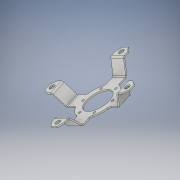
# Autodesk Inventor part: Actividad 4.1_Emily_Rojas
Saved by Autodesk Inventor 2019 (Build 230136000, 136)
## iProperties
Created: 2019-05-23
Part Number: Actividad 4.1_Emily_Rojas
Material: Generic
Document SubType Name: Sheet Metal
Designer: Emily Rojas
Density: 1 g/cm^3
Sheet Metal Rule: Default
Appearance: Default
Author: Emily Rojas
Autodesk Inventor part; units mm, degrees
ref_plane "YZ Plane" through (0, 0, 0) normal (1, 0, 0) x (0, 1, 0)
ref_plane "XZ Plane" through (0, 0, 0) normal (0, 1, 0) x (-1, 0, 0)
ref_plane "XY Plane" through (0, 0, 0) normal (0, 0, 1) x (1, 0, 0)
sketch "Sketch1" plane through (0, 0, 0) normal (0, 1, 0) x (-1, 0, 0)
  circle A0 centre (0, 0) radius 10
  circle A1 centre (12.5, 0.022) radius 1
  circle A2 centre (6.231, 10.8363) radius 1
  circle A3 centre (-6.269, 10.8143) radius 1
  circle A4 centre (-12.5, -0.022) radius 1
  circle A5 centre (-6.231, -10.8363) radius 1
  circle A6 centre (6.269, -10.8143) radius 1
  line L0 (-12.4513, 1.1023) -> (-12.5238, 0.9777)
  line L1 (-12.5238, 0.9777) -> (-38.4555, 16.0624)
  line L2 (-38.4555, 16.0624) -> (-33.0451, 25.3632)
  line L3 (-33.0451, 25.3632) -> (-7.1134, 10.2786)
  line L4 (-0.9777, -12.5238) -> (-16.0624, -38.4555)
  line L5 (-25.3632, -33.0451) -> (-10.2786, -7.1134)
  line L6 (-16.0624, -38.4555) -> (-25.3632, -33.0451)
  line L7 (12.5238, -0.9777) -> (38.4555, -16.0624)
  line L8 (33.0451, -25.3632) -> (7.1134, -10.2786)
  line L9 (38.4555, -16.0624) -> (33.0451, -25.3632)
  line L10 (0.9777, 12.5238) -> (16.0624, 38.4555)
  line L11 (25.3632, 33.0451) -> (10.2786, 7.1134)
  line L12 (16.0624, 38.4555) -> (25.3632, 33.0451)
  circle A7 centre (-18.7015, -32.2927) radius 2
  circle A8 centre (32.2927, -18.7015) radius 2
  circle A9 centre (18.7015, 32.2927) radius 2
  circle A10 centre (-32.2927, 18.7015) radius 2
  arc A11 (-2.3138, -14.8205) -> (9.458, -11.6424) centre (0, 0) ccw
  arc A12 (14.8205, -2.3138) -> (11.6424, 9.458) centre (0, 0) ccw
  arc A13 (2.3138, 14.8205) -> (-9.458, 11.6424) centre (0, 0) ccw
  arc A14 (-14.8205, 2.3138) -> (-11.6424, -9.458) centre (0, 0) ccw
  arc A15 (12.4617, -0.9773) -> (12.4644, -0.9432) centre (0, 0) ccw
  arc A16 (6.9816, -10.3686) -> (7.1134, -10.2786) centre (0, 0) ccw
  arc A17 (-6.9816, 10.3686) -> (-7.1134, 10.2786) centre (0, 0) ccw
  arc A18 (-12.4513, 1.1023) -> (-12.4617, 0.9773) centre (0, 0) ccw
  dimension "d3" = 2
  dimension "d0" = 20
  dimension "d6" = 360
  dimension "d8" = 30
  dimension "d11" = 360
  dimension "d13" = 4
  dimension "d14" = 5.38
  dimension "d15" = 4
  dimension "d16" = 5.38
  dimension "d19" = 360
  measures "d0" diameter of A0
  measures "d8" distance between parallel lines of L2 L0
  measures "d13" diameter of A7
  measures "d14" distance from line of L4 A7.centre
  measures "d15" distance from line of L6 A7.centre
  measures "d16" distance from line of L5 A7.centre
extrude "Plate1" add sketch "Sketch1" along normal blind 1
fillet "Corner Round1" radius 2 8 edges at (14.8205, 0.5, 2.3138) (11.6424, 0.5, -9.458) (9.458, 0.5, 11.6424) (-2.3138, 0.5, 14.8205) (-11.6424, 0.5, 9.458) (-14.8205, 0.5, -2.3138) (-9.458, 0.5, -11.6424) (2.3138, 0.5, -14.8205)
sketch "Sketch2" plane through (0, 1, 0) normal (0, 1, 0) x (1, 0, 0)
  line L0 (-25.3632, -33.0451) -> (-12.306, -10.5986) projected
  line L1 (-15.5823, -16.2309) -> (-6.2636, -21.6106)
  line L2 (-2.9702, -15.949) -> (-16.0624, -38.4555) projected
  line L3 (10.5986, -12.306) -> (33.0451, -25.3632) projected
  line L4 (16.2309, -15.5823) -> (21.6106, -6.2636)
  line L5 (38.4555, -16.0624) -> (15.949, -2.9702) projected
  line L6 (25.3632, 33.0451) -> (12.306, 10.5986) projected
  line L7 (15.5823, 16.2309) -> (6.2636, 21.6106)
  line L8 (16.0624, 38.4555) -> (2.9702, 15.949) projected
  line L9 (-10.5986, 12.306) -> (-33.0451, 25.3632) projected
  line L10 (-16.2309, 15.5823) -> (-21.6106, 6.2636)
  line L11 (-38.4555, 16.0624) -> (-15.949, 2.9702) projected
  arc A0 (-21.6106, 6.2636) -> (-15.5823, -16.2309) centre (0, 0) ccw
  arc A1 (-6.2636, -21.6106) -> (16.2309, -15.5823) centre (0, 0) ccw
  arc A2 (21.6106, -6.2636) -> (15.5823, 16.2309) centre (0, 0) ccw
  arc A3 (6.2636, 21.6106) -> (-16.2309, 15.5823) centre (0, 0) ccw
  constraints: 8 end point, 8 point on circle, 8 point on line, 4 centre point, 1 coincident
fold "Fold1" angle 60 bend radius 1 thickness 1 k factor 0.44 line from (-16.2309, 1, -15.5823) to (-21.6106, 1, -6.2636) line at bend centre moving side (0.8660444, 0, 0.4999671) folds toward (0, 1, 0)
sketch "Sketch3" plane through (-14.9991, 24.4453, 9.0047) normal (-0.7500165, 0.5, -0.4329842) x (-0.5013925, -0.0028562, 0.8652152)
  circle A0 centre (-15.2796, -5.4521) radius 10 projected
  arc A1 (-37.1091, -10.9041) -> (-37.1446, -0.1441) centre (-15.2796, -5.4521) ccw
  line L0 (-30.5592, -10.9041) -> (-56.5967, -10.9041) projected
  line L1 (-37.1091, -10.9041) -> (-37.1446, -0.1441)
  line L2 (-56.5967, -0.1441) -> (-30.6287, -0.1441) projected
  point P0 (-15.2416, -16.9767)
  dimension "d30" = 45
  constraints: 2 end point, 2 point on circle, 2 point on line, 1 centre point, 1 coincident
  measures "d30" diameter of A1
fold "Fold2" angle 60 bend radius 1 thickness 1 k factor 0.44 line from (-1.0966, 15.1081, -25.8596) to (3.5628, 24.4266, -23.1698) line at bend centre moving side (0.4999671, 0, -0.8660444) folds toward (-0.7500165, 0.5, -0.4329842)
sketch "Sketch4" plane through (-14.9991, 24.4453, 9.0047) normal (-0.7500165, 0.5, -0.4329842) x (-0.5013925, -0.0028562, 0.8652152)
  circle A0 centre (-15.2796, -5.4521) radius 10 projected
  arc A1 (-20.7317, 16.3774) -> (-9.9717, 16.4129) centre (-15.2796, -5.4521) ccw
  line L0 (-9.9717, 35.865) -> (-9.9717, 9.897) projected
  line L1 (-9.9717, 16.4129) -> (-20.7317, 16.3774)
  line L2 (-20.7317, 9.8276) -> (-20.7317, 35.865) projected
  point P0 (-15.2416, -16.9767)
  dimension "d37" = 45
  constraints: 2 end point, 2 point on circle, 2 point on line, 1 centre point, 1 coincident
  measures "d37" diameter of A1
fold "Fold3" angle 60 bend radius 1 thickness 1 k factor 0.44 line from (-2.9193, 38.6877, 4.5269) to (2.4604, 38.6877, -4.7918) line at bend centre moving side (-0.4330222, -0.8660254, -0.2499835) folds toward (-0.7500165, 0.5, -0.4329842)
sketch "Sketch5" plane through (-34.9831, 38.8407, 27.5325) normal (0, 1, 0) x (0.8643908, 0, 0.5028206)
  circle A0 centre (-5.4521, 41.3171) radius 10 projected
  arc A1 (0, 19.4876) -> (-10.76, 19.4521) centre (-5.4521, 41.3171) ccw
  line L0 (-10.76, 25.968) -> (-10.76, 0) projected
  line L1 (-10.76, 19.4521) -> (0, 19.4876)
  line L2 (0, 0) -> (0, 26.0374) projected
  point P0 (16.3951, 41.3891)
  dimension "d44" = 45
  constraints: 2 end point, 2 point on circle, 2 point on line, 1 centre point, 1 coincident
  measures "d44" diameter of A1
fold "Fold4" angle 60 bend radius 1 thickness 1 k factor 0.44 line from (-34.503, 38.8407, 5.308) to (-25.1843, 38.8407, 10.6876) line at bend centre moving side (0.4999671, 0, -0.8660444) folds toward (0, 1, 0)
sketch "Sketch7" plane through (-44.284, 37.8407, 22.1222) normal (0, -1, 0) x (0.8643908, 0, 0.5028206)
  line L0 (10.76, 0) -> (10.76, -18.7336) projected
  line L1 (10.76, -8) -> (0, -8)
  line L2 (0, 0) -> (10.76, 0) projected
  line L3 (0, -18.6981) -> (0, 0) projected
  point P0 (27.1551, -41.3891)
  dimension "d51" = 8
  constraints: 2 end point, 2 point on line, 1 horizontal
  measures "d51" distance between parallel lines of L2 L1
fold "Fold5" angle 60 bend radius 1 thickness 1 k factor 0.44 line from (-30.9605, 37.8407, 20.6174) to (-40.2614, 37.8407, 15.2071) line at bend centre moving side (0.5028206, 0, -0.8643908) folds toward (0, -1, 0)
sketch "Sketch8" plane through (-44.0486, 28.7786, -13.0295) normal (-0.7505334, -0.4975244, -0.4349357) x (-0.5028115, 0.0028586, 0.8643914)
  line L0 (0, 10.7336) -> (-10.76, 10.7336)
  line L1 (-10.76, 18.7336) -> (0, 18.7336) projected
  line L2 (-10.76, 0.0355) -> (-10.76, 18.7336) projected
  line L3 (0, 18.7336) -> (0, 0) projected
  point P0 (-10.9678, -47.1399)
  dimension "d58" = 8
  constraints: 2 end point, 2 point on line, 1 horizontal
  measures "d58" distance between parallel lines of L1 L0
fold "Fold6" angle 60 bend radius 1 thickness 1 k factor 0.44 line from (-48.6513, 38.0895, -15.7377) to (-43.241, 38.0587, -25.0385) line at bend centre moving side (0.4288125, -0.8674453, 0.2523064) folds toward (-0.7505334, -0.4975244, -0.4349357)
sketch "Sketch9" plane through (-14.7051, 21.998, -39.3814) normal (0.0621417, -0.2487704, -0.966567) x (-0.9022703, -0.4280055, 0.05215)
  line L0 (8, 0) -> (8, -10.76)
  line L1 (0, -10.76) -> (0, 0) projected
  line L2 (18.6981, -10.76) -> (0, -10.76) projected
  line L3 (0, 0) -> (18.7336, 0) projected
  point P0 (-1.7989, -35.2744)
  dimension "d65" = 8
  constraints: 2 end point, 2 point on line, 1 vertical
  measures "d65" distance between parallel lines of L1 L0
fold "Fold7" angle 60 bend radius 1 thickness 1 k factor 0.44 line from (-21.9232, 18.574, -38.9642) to (-17.3323, 9.225, -36.2629) line at bend centre moving side (-0.9022703, -0.4280055, 0.05215) folds toward (0.0621417, -0.2487704, -0.966567)
sketch "Sketch10" plane through (-29.6185, -17.8413, -39.4621) normal (0.4023205, -0.8768526, -0.2631878) x (0.9020855, 0.428722, -0.0493889)
  line L0 (0, 10.7336) -> (-10.76, 10.7336)
  line L1 (-10.76, 18.7336) -> (0, 18.7336) projected
  line L2 (-10.76, 0.0355) -> (-10.76, 18.7336) projected
  line L3 (0, 18.7336) -> (0, 0) projected
  point P0 (32.4184, 38.7642)
  dimension "d72" = 8
  constraints: 2 end point, 2 point on line, 1 horizontal
  measures "d72" distance between parallel lines of L1 L0
fold "Fold8" angle 60 bend radius 1 thickness 1 k factor 0.44 line from (-27.9425, -20.1763, -29.1205) to (-37.649, -24.7894, -28.589) line at bend centre moving side (-0.1561412, 0.2175477, -0.9634796) folds toward (0.4023205, -0.8768526, -0.2631878)
chamfer "Corner Chamfer1" distance 4 distance2 3 1 edges at (-38.1127, -5.884, -90.5016) measured on face at (-38.0346, -5.9928, -90.0199)
chamfer "Corner Chamfer2" distance 4 distance2 3 1 edges at (-4.0754, -1.8474, -52.2504) measured on face at (-4.5271, -2.0605, -52.2254)
chamfer "Corner Chamfer3" distance 4 distance2 3 1 edges at (-36.601, -26.0913, -20.7496) measured on face at (-36.6791, -25.9826, -21.2313)
chamfer "Corner Chamfer4" distance 4 distance2 3 1 edges at (-70.6383, -30.1279, -59.0008) measured on face at (-70.1867, -29.9148, -59.0258)
chamfer "Corner Chamfer5" distance 3 distance2 4 1 edges at (-68.9705, -32.4417, -48.6257) measured on face at (-69.048, -32.3342, -49.1078)
chamfer "Corner Chamfer6" distance 3 distance2 4 1 edges at (-26.8946, -21.4783, -21.281) measured on face at (-27.3456, -21.6926, -21.2563)
chamfer "Corner Chamfer7" distance 3 distance2 4 1 edges at (-5.7678, 0.5203, -62.6094) measured on face at (-5.6892, 0.4103, -62.128)
chamfer "Corner Chamfer8" distance 3 distance2 4 1 edges at (-47.8437, -10.4431, -89.954) measured on face at (-47.3915, -10.2312, -89.9795)
equation "\"d21\" = Thickness"
equation "\"d24\" = BendReliefWidth"
equation "\"d25\" = BendReliefDepth"
equation "\"d26\" = MinimumRemnant"
equation "\"d27\" = TransitionRadius"
equation "\"d29\" = BendRadius"
equation "\"d31\" = BendReliefWidth"
equation "\"d32\" = BendReliefDepth"
equation "\"d33\" = MinimumRemnant"
equation "\"d34\" = TransitionRadius"
equation "\"d36\" = BendRadius"
equation "\"d38\" = BendReliefWidth"
equation "\"d39\" = BendReliefDepth"
equation "\"d40\" = MinimumRemnant"
equation "\"d41\" = TransitionRadius"
equation "\"d43\" = BendRadius"
equation "\"d45\" = BendReliefWidth"
equation "\"d46\" = BendReliefDepth"
equation "\"d47\" = MinimumRemnant"
equation "\"d48\" = TransitionRadius"
equation "\"d50\" = BendRadius"
equation "\"d52\" = BendReliefWidth"
equation "\"d53\" = BendReliefDepth"
equation "\"d54\" = MinimumRemnant"
equation "\"d55\" = TransitionRadius"
equation "\"d57\" = BendRadius"
equation "\"d59\" = BendReliefWidth"
equation "\"d60\" = BendReliefDepth"
equation "\"d61\" = MinimumRemnant"
equation "\"d62\" = TransitionRadius"
equation "\"d64\" = BendRadius"
equation "\"d66\" = BendReliefWidth"
equation "\"d67\" = BendReliefDepth"
equation "\"d68\" = MinimumRemnant"
equation "\"d69\" = TransitionRadius"
equation "\"d71\" = BendRadius"
equation "\"d73\" = BendReliefWidth"
equation "\"d74\" = BendReliefDepth"
equation "\"d75\" = MinimumRemnant"
equation "\"d76\" = TransitionRadius"
equation "\"d78\" = BendRadius"
equation "\"BendRadius\" = Thickness"
equation "\"BendReliefWidth\" = Thickness"
equation "\"BendReliefDepth\" = 0.5 * Thickness"
equation "\"CornerReliefSize\" = 4 * Thickness"
equation "\"MinimumRemnant\" = 2 * Thickness"
equation "\"TransitionRadius\" = BendRadius"
equation "\"JacobiRadiusSize\" = Thickness"
equation "\"GapSize\" = Thickness"
equation "\"Thickness\" = 1"
body "Solid1"
